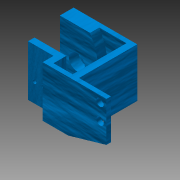
# Autodesk Inventor part: Encoder Mount v2
Saved by Autodesk Inventor 2015 (Build 190159000, 159)
## iProperties
Created: 2015-04-22
Part Number: Encoder Mount v2
Material: PLA Plastic
Document SubType Name: Modeling
Designer: Kyle
Density: 1 g/cm^3
Appearance: Generic(1)
Author: Kyle
Autodesk Inventor part; units mm, degrees
ref_plane "YZ Plane" through (0, 0, 0) normal (1, 0, 0) x (0, 1, 0)
ref_plane "XZ Plane" through (0, 0, 0) normal (0, 1, 0) x (-1, 0, 0)
ref_plane "XY Plane" through (0, 0, 0) normal (0, 0, 1) x (1, 0, 0)
sketch "Sketch1" plane through (0, 0, 0) normal (0, 1, 0) x (-1, 0, 0)
  line L0 (-3.1474, 0) -> (12.0926, 0)
  line L1 (12.0926, 0) -> (12.0926, -23.222)
  line L2 (12.0926, -23.222) -> (34.9526, -23.222)
  line L3 (34.9526, -25) -> (9.5526, -25)
  line L4 (9.5526, -25) -> (9.5526, -1.778)
  line L5 (9.5526, -1.778) -> (-3.1474, -1.778)
  line L6 (-3.1474, -1.778) -> (-3.1474, 0)
  line L7 (34.9526, -25) -> (34.9526, -23.222)
  dimension "d1" = 1.778
  dimension "d2" = 25
  dimension "d3" = 1.778
  dimension "d5" = 25.4
  dimension "d6" = 2.54
  dimension "d26" = 15.24
  constraints: 16 end point, 5 perpendicular, 1 horizontal, 1 vertical
  measures "d1" distance of L5.end L0.start
  measures "d2" distance between parallel lines of L0 L3
  measures "d3" distance between parallel lines of L3 L2
  measures "d5" distance of L3.start L3.end
  measures "d6" distance between parallel lines of L1 L4
  measures "d26" distance of L0.start L0.end
extrude "Extrusion1" add sketch "Sketch1" along normal mid plane 25.4
sketch "Sketch2" plane through (-34.9526, 12.7, -23.222) normal (0, 0, 1) x (1, 0, 0)
  arc A0 (12.0273, -25.4) -> (12.0273, 0) centre (-9.5066, -12.7) ccw
  line L0 (0, 0) -> (12.0273, 0)
  line L1 (12.1267, -25.23) -> (0, -25.23)
  line L2 (0, -25.23) -> (0, 0)
  line L3 (11.8723, 0) -> (11.8723, -12.7) construction
  line L4 (11.8723, -12.7) -> (11.8723, -25.4) construction
  line L5 (22.86, -25.4) -> (0, -25.4) construction
  line L6 (11.8723, -12.7) -> (-9.5066, -12.7) construction
  line L7 (0, 0) -> (0, -25.4) construction
  point P0 (34.9526, -12.7)
  dimension "d9" = 50
  constraints: 12 end point, 4 point on line, 3 point on circle, 1 centre point, 1 coincident, 1 collinear, 1 horizontal, 1 parallel, 1 perpendicular, 1 vertical
  measures "d9" diameter of A0
extrude "Extrusion2" add sketch "Sketch2" along normal blind 3.7
sketch "Sketch3" plane through (3.1474, 12.7, -1.778) normal (0, 0, -1) x (-1, 0, 0)
  line L0 (0, -25.4) -> (0, 0) projected
  line L1 (0, -15.8818) -> (33.02, -25.4)
  line L2 (38.1, -25.4) -> (12.7, -25.4) projected
  line L3 (0, -25.4) -> (0, -15.8818)
  line L4 (0, -25.4) -> (33.02, -25.4)
  point P0 (3.1474, -12.7)
  point P1 (0, 0)
  dimension "d12" = 73.92
  dimension "d13" = 33.02
  constraints: 6 end point, 1 horizontal, 1 point on line, 1 vertical, 2 other
  measures "d12" angle to the sketch y axis of L1
  measures "d13" distance of L1.end L3.start
extrude "Extrusion3" cut sketch "Sketch3" along normal mid plane 76.2
sketch "Sketch4" plane through (3.1474, 12.7, -1.778) normal (0, 0, -1) x (-1, 0, 0)
  line L0 (0, -15.8818) -> (0, -8.9488) construction
  line L1 (0, 0) -> (0, -15.8818) construction
  line L2 (2.54, -8.9488) -> (2.54, -2.4488) construction
  line L3 (0, -8.9488) -> (2.54, -8.9488) construction
  point P0 (3.1474, -12.7)
  dimension "d16" = 6.933
  dimension "d17" = 2.54
  dimension "d18" = 6.5
  constraints: 6 end point, 1 horizontal, 1 vertical, 2 other
  measures "d16" distance of L0.start L0.end
  measures "d17" distance of L0.end L2.start
  measures "d18" distance of L2.start L2.end
hole "Hole1" at (0.6074, 3.7512, -1.778) at (0.6074, 10.2512, -1.778) direction (0, 0, 1) diameter 3 end through all
sketch "Sketch5" plane through (-34.9526, 12.7, -19.522) normal (0, 0, 1) x (1, 0, 0)
  circle A0 centre (6.8106, -12.7) radius 3.175
  point P0 (34.9526, -12.7)
  dimension "d28" = 6.35
  constraints: 1 centre point
  measures "d28" diameter of A0
extrude "Extrusion4" cut sketch "Sketch5" against normal blind 3.81
sketch "Sketch6" plane through (-28.1421, 0, -23.332) normal (0, 0, 1) x (1, 0, 0)
  line L0 (-0.0036, 0) -> (1.7744, 0)
  line L1 (-0.0036, 0) -> (-1.7816, 0)
  point P0 (28.1421, 0)
  dimension "d31" = 1.778
  constraints: 4 end point, 2 horizontal, 1 collinear
  measures "d31" distance of L0.start L0.end
hole "Hole2" at (-29.9236, 0, -23.332) at (-26.3676, 0, -23.332) direction (0, 0, -1) diameter 1.5 end through all
sketch "Sketch7" plane through (-12.0926, 12.7, -23.222) normal (-1, 0, 0) x (0, 0, 1)
  line L0 (23.222, -20.2748) -> (21.444, -20.2748)
  line L1 (21.444, -20.2748) -> (21.444, 0)
  line L2 (21.444, 0) -> (23.222, 0)
  line L3 (23.222, 0) -> (23.222, -20.2748)
  point P0 (23.222, -12.7)
  constraints: 8 end point, 2 parallel, 1 horizontal, 1 perpendicular
extrude "Extrusion5" add sketch "Sketch7" along normal blind 10.16
sketch "Sketch8" plane through (-12.0926, -7.5748, -1.778) normal (0, 0, -1) x (-1, 0, 0)
  line L0 (0, 20.2748) -> (10.16, 20.2748) projected
  line L1 (10.16, 0) -> (7.62, 0)
  line L2 (7.62, 0) -> (7.62, 20.2748)
  line L3 (7.62, 20.2748) -> (10.16, 20.2748)
  line L4 (10.16, 20.2748) -> (10.16, 0)
  point P0 (-12.0926, 7.5748)
  dimension "d43" = 2.54
  constraints: 8 end point, 2 parallel, 1 horizontal, 1 perpendicular, 1 point on line
  measures "d43" distance of L1.start L1.end
extrude "Extrusion6" add sketch "Sketch8" along normal blind 5.08
sketch "Sketch9" plane through (-22.2526, 12.7, -23.222) normal (-1, 0, 0) x (0, 0, 1)
  line L0 (0, -20.2748) -> (21.444, -20.2748) projected
  line L1 (16.364, 0) -> (18.904, 0)
  line L2 (18.904, 0) -> (18.904, -20.2748)
  line L3 (18.904, -20.2748) -> (16.364, -20.2748)
  line L4 (16.364, -20.2748) -> (16.364, 0)
  point P0 (23.222, -12.7)
  dimension "d44" = 2.54
  constraints: 8 end point, 2 parallel, 1 horizontal, 1 perpendicular, 1 point on line
  measures "d44" distance of L1.start L1.end
extrude "Extrusion7" add sketch "Sketch9" along normal blind 10.16
sketch "Sketch10" plane through (-12.0926, -7.5748, -6.858) normal (0, 0, -1) x (-1, 0, 0)
  line L0 (16.002, 20.2748) -> (16.002, 7.5748)
  line L1 (16.002, 7.5748) -> (14.224, 7.5748)
  line L2 (7.62, 20.2748) -> (16.002, 20.2748) construction
  line L3 (7.62, 20.2748) -> (7.62, 0) construction
  line L4 (16.002, 7.5748) -> (17.78, 7.5748)
  point P0 (-12.0926, 7.5748)
  point P1 (20.32, 20.2748)
  dimension "d47" = 1.778
  dimension "d48" = 8.382
  dimension "d49" = 12.7
  constraints: 8 end point, 2 perpendicular, 1 collinear, 1 horizontal, 1 vertical
  measures "d47" distance of L0.end L1.end
  measures "d48" distance of L2.start L0.start
  measures "d49" distance of L0.start L0.end
hole "Hole3" at (-26.3166, 0, -6.858) at (-29.8726, 0, -6.858) direction (0, 0, 1) diameter 1.5 end through all
body "Solid1"
